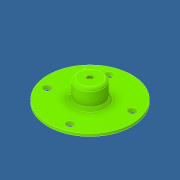
# Autodesk Inventor part: OberArmMagnet
Saved by Autodesk Inventor 2016 (Build 200138000, 138)
## iProperties
Created: 2015-09-18
Part Number: OberArmMagnet
Material: ABS-Kunststoff
Document SubType Name: Modeling
Designer: 4ndreas
Density: 1.06 g/cm^3
Appearance: Glatt - grün
Mass: 28.5695 g
Surface Area: 179.385 cm^2
Volume: 26.9523 cm^3
Author: 4ndreas
Autodesk Inventor part; units mm, degrees
ref_plane "YZ Plane" through (0, 0, 0) normal (1, 0, 0) x (0, 1, 0)
ref_plane "XZ Plane" through (0, 0, 0) normal (0, 1, 0) x (-1, 0, 0)
ref_plane "XY Plane" through (0, 0, 0) normal (0, 0, 1) x (1, 0, 0)
sketch "Skizze1" plane through (0, 0, 0) normal (0, 0, 1) x (1, 0, 0)
  circle A0 centre (-35.2385, -12.8258) radius 2.1 projected
  circle A1 centre (-12.8258, 35.2385) radius 2.1 projected
  circle A2 centre (12.8258, -35.2385) radius 2.1 projected
  circle A3 centre (35.2385, 12.8258) radius 2.1 projected
  circle A4 centre (0, 0) radius 25 projected
  circle A5 centre (0, 0) radius 45 projected
  circle A6 centre (0, 0) radius 47.5 projected
  circle A7 centre (0, 0) radius 8.4675
  point P0 (0, 0)
  constraints: 1 centre point, 1 coincident
extrude "Extrusion1" add sketch "Skizze1" along normal blind 3 contours A4 | A5 | A6 | A7
sketch "Skizze2" plane through (0, 0, 3) normal (0, 0, 1) x (1, 0, 0)
  circle A0 centre (0, 0) radius 15
  dimension "d2" = 30
  constraints: 1 centre point, 1 coincident
  measures "d2" diameter of A0
extrude "Extrusion2" add sketch "Skizze2" along normal blind 21
sketch "Skizze3" plane through (0, 0, 24) normal (0, 0, 1) x (1, 0, 0)
  circle A0 centre (0, 0) radius 3
  dimension "d7" = 6
  constraints: 1 centre point, 1 coincident
  measures "d7" diameter of A0
extrude "Extrusion3" cut sketch "Skizze3" against normal blind 2.5
sketch "Skizze4" plane through (0, 0, 0) normal (0, 0, -1) x (-1, 0, 0)
  circle A0 centre (0, 0) radius 15 projected
  circle A1 centre (0, 0) radius 11
  dimension "d8" = 4
  constraints: 1 centre point, 1 coincident
  measures "d8" radial gap between concentric circles of A0 A1
extrude "Extrusion4" cut sketch "Skizze4" against normal blind 20 contours A1
sketch "Skizze5" plane through (0, 0, 0) normal (0, 0, -1) x (-1, 0, 0)
  circle A0 centre (0, 0) radius 11 projected
  circle A1 centre (-35.2385, 12.8258) radius 2.1 projected
  circle A2 centre (-12.8258, -35.2385) radius 2.1 projected
  circle A3 centre (12.8258, 35.2385) radius 2.1 projected
  circle A4 centre (35.2385, -12.8258) radius 2.1 projected
  circle A5 centre (0, 0) radius 47.5 projected
  line L0 (6, -9.2195) -> (6, 9.2195)
  dimension "d11" = 6
  constraints: 2 end point, 2 point on circle, 1 vertical
  measures "d11" distance from line of L0 point (0, 0)
extrude "Extrusion5" add sketch "Skizze5" against normal up to surface (20 mm away) contours A0 L0 picked at (7.6667, 0)
sketch "Skizze6" plane through (-6, -9.2195, 0) normal (1, 0, 0) x (0, 0, -1)
  line L0 (-20, 0) -> (-20, 18.4391) projected
  line L1 (0, 0) -> (-20, 0) projected
  line L2 (0, 18.4391) -> (0, 0) projected
  line L3 (-20, 18.4391) -> (0, 18.4391) projected
  line L4 (-3, -5.7805) -> (-3, 24.2195) projected
  line L5 (-3, 19.9453) -> (-3, 24.1453) projected
  line L6 (-3, -28.1189) -> (-3, -23.9189) projected
  line L7 (-3, 42.358) -> (-3, 46.558) projected
  line L8 (-3, -5.7062) -> (-3, -1.5062) projected
  line L9 (-3, 56.7195) -> (-3, -38.2805) projected
  line L10 (-3, 0) -> (-20, 0)
  line L11 (-20, 0) -> (-20, 18.4391)
  line L12 (-20, 18.4391) -> (-3, 18.4391)
  line L13 (-3, 18.4391) -> (-3, 0)
  point P0 (0, 9.2195)
  constraints: 8 end point, 3 point on line, 2 parallel, 1 collinear, 1 horizontal, 1 perpendicular
extrude "Extrusion6" cut sketch "Skizze6" against normal blind 20 contours L0 L3 L4 L1
sketch "Skizze7" plane through (0, 0, 20) normal (0, 0, -1) x (-1, 0, 0)
  arc A0 (6, 9.2195) -> (6, -9.2195) centre (0, 0) ccw projected
  line L0 (6, -9.2195) -> (11.8322, -9.2195) projected
  arc A1 (11.8322, -9.2195) -> (11.8322, 9.2195) centre (0, 0) ccw projected
  line L1 (6, 9.2195) -> (11.8322, 9.2195) projected
  line L2 (11.8322, 9.2195) -> (11.8322, -9.2195)
  constraints: 2 end point, 1 vertical
extrude "Extrusion7" cut sketch "Skizze7" against normal blind 20 contours A1 L2
chamfer "Fase1" distance 3 angle 45 1 edges at (15, 0, 3)
chamfer "Fase2" distance 2.5 angle 45 4 edges at (-14.9258, 35.2385, 3) (33.1385, 12.8258, 3) (10.7258, -35.2385, 3) (-37.3385, -12.8258, 3)
fillet "Rundung1" radius 3 2 edges at (-10.7298, 9.2195, 3) (-10.7298, -9.2195, 3)
chamfer "Fase3" distance 2 angle 45 2 edges at (-8.9161, 9.2195, 20) (-8.9161, -9.2195, 20)
fillet "Rundung2" radius 3 2 edges at (-8.9161, 9.2195, 18) (-8.9161, -9.2195, 18)
fillet "Rundung3" radius 3 1 edges at (15, 0, 24)
